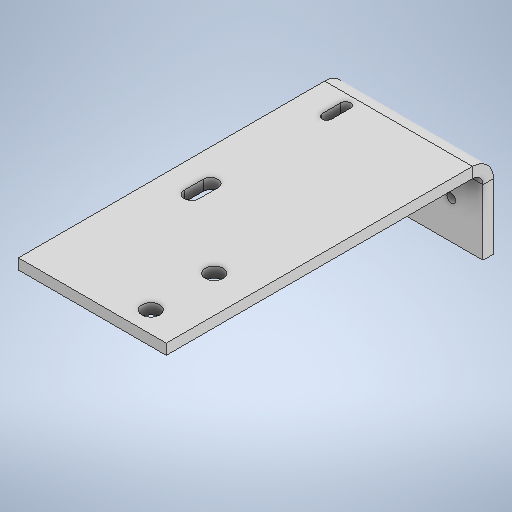
# Autodesk Inventor part: ER_Halterung_Kantensensor
Saved by Autodesk Inventor 2025.1 (Build 291241000, 241)
## iProperties
Created: 2025-06-20
Part Number: ER_Halterung_Kantensensor
Material: Generic
Document SubType Name: Sheet Metal
Designer: Erik
Density: 1 g/cm^3
Sheet Metal Rule: Default_mm
Appearance: Default
Author: Erik
Autodesk Inventor part; units mm, degrees
ref_plane "YZ Plane" through (0, 0, 0) normal (1, 0, 0) x (0, 1, 0)
ref_plane "XZ Plane" through (0, 0, 0) normal (0, 1, 0) x (-1, 0, 0)
ref_plane "XY Plane" through (0, 0, 0) normal (0, 0, 1) x (1, 0, 0)
sketch "Sketch1" plane through (0, 0, 0) normal (0, 1, 0) x (-1, 0, 0)
  line L0 (0, 0) -> (70, 0)
  line L1 (70, 0) -> (70, -150)
  line L2 (70, -150) -> (0, -150)
  line L3 (0, -150) -> (0, 0)
  dimension "d0" = 70
  dimension "d1" = 150
  measures "d0" distance of L1.end L2.end
  measures "d1" distance of L0.end L1.end
extrude "Plate1" add sketch "Sketch1" along normal blind 5
sketch "Sketch2" plane through (0, 0, -150) normal (0, 0, -1) x (-1, 0, 0)
  line L0 (70, 5) -> (0, 5)
  line L1 (0, 5) -> (70, 5)
  line L2 (70, 5) -> (70, -36)
  line L3 (70, -36) -> (0, -36)
  line L4 (0, -36) -> (0, 5)
  point P0 (0, 0)
  dimension "d3" = 70
  dimension "d4" = 41
  measures "d3" distance of L2.end L3.end
  measures "d4" distance of L1.end L2.end
sheet face with bend "Face2" sketch "Sketch2" thickness 5 toward (0, 0, -1) bend radius 5 relief straight relief width 5 relief depth 2.5
bend "Bend1"
sketch "Sketch3" plane through (0, 0, -155) normal (0, 0, -1) x (-1, 0, 0)
  line L0 (70, -36) -> (0, -36) projected
  line L1 (70, -5) -> (70, -36) projected
  point P0 (0, 0)
  point P1 (45, -18)
  point P2 (15, -18)
  dimension "d10" = 18
  dimension "d11" = 18
  dimension "d19" = 25
  dimension "d20" = 30
  measures "d10" distance from line of L0 point (45, -18)
  measures "d11" distance from line of L0 point (15, -18)
  measures "d19" distance from line of L1 point (45, -18)
  measures "d20" distance of point (45, -18) point (15, -18)
hole "Hole1" at (-45, -18, -155) at (-15, -18, -155) direction (0, 0, 1) diameter 4.134 depth 5 tip angle 118 thread size "M5x0.8" class "6H" standard "ISO Metric profile"
sketch "Sketch4" plane through (0, 5, 0) normal (0, 1, 0) x (1, 0, 0)
  line L0 (-70, 145) -> (0, 145) projected
  line L1 (-55, 145) -> (-55, 0) construction
  line L2 (-70, 0) -> (0, 0) projected
  line L3 (-70, 0) -> (-70, 145) projected
  line L4 (-57.25, 131) -> (-52.75, 131)
  line L5 (-52.75, 131) -> (-52.75, 140)
  line L6 (-52.75, 140) -> (-57.25, 140)
  line L7 (-57.25, 140) -> (-57.25, 131)
  line L8 (-57.25, 131) -> (-52.75, 140) construction
  line L9 (-52.75, 131) -> (-57.25, 140) construction
  arc A0 (-52.75, 140) -> (-57.25, 140) centre (-55, 140) ccw
  arc A1 (-57.25, 131) -> (-52.75, 131) centre (-55, 131) ccw
  line L10 (-55, 140) -> (-51.5, 76.0958) construction
  line L11 (-55, 140) -> (9, 140) construction
  line L12 (-55, 131) -> (-51.5, 67.0958) construction
  line L13 (-55, 131) -> (9, 131) construction
  line L14 (-58.5, 67) -> (-51.5, 67)
  line L15 (-51.5, 67) -> (-51.5, 76)
  line L16 (-51.5, 76) -> (-58.5, 76)
  line L17 (-58.5, 76) -> (-58.5, 67)
  line L18 (-58.5, 67) -> (-51.5, 76) construction
  line L19 (-51.5, 67) -> (-58.5, 76) construction
  arc A2 (-51.5, 76) -> (-58.5, 76) centre (-55, 76) ccw
  arc A3 (-58.5, 67) -> (-51.5, 67) centre (-55, 67) ccw
  point P0 (-70, 72.5)
  point P1 (-55, 135.5)
  point P2 (-55, 71.5)
  dimension "d21" = 15
  dimension "d22" = 4.5
  dimension "d23" = 9
  dimension "d25" = 5
  dimension "d32" = 64
  dimension "d34" = 64
  dimension "d36" = 7
  dimension "d37" = 9
  dimension "d40" = 64
  constraints: 34 end point, 8 midpoint, 8 point on circle, 8 tangent, 6 point on line, 4 centre point, 4 horizontal, 4 parallel, 2 equal length, 2 perpendicular, 1 vertical
  measures "d21" distance from line of point (-70, 72.5) L1
  measures "d22" distance between parallel lines of L5 L7
  measures "d23" distance of point (-55, 140) point (-55, 131)
  measures "d25" distance from line of L0 point (-55, 140)
  measures "d32" distance of L10.start L10.end
  measures "d34" distance of L12.start L12.end
  measures "d36" distance of L16.end L15.end
  measures "d37" distance between parallel lines of L16 L14
  measures "d40" distance of point (-55, 140) point (-55, 76)
extrude "Extrusion1" cut sketch "Sketch4" against normal up to surface (5 mm away)
sketch "Sketch5" plane through (0, 5, 0) normal (0, 1, 0) x (1, 0, 0)
  line L0 (-70, 0) -> (-70, 145) projected
  line L1 (0, 0) -> (-70, 0) projected
  point P0 (-17.3, 40)
  point P1 (-17.3, 10)
  dimension "d41" = 52.7
  dimension "d42" = 52.7
  dimension "d50" = 30
  dimension "d51" = 10
  measures "d41" distance from line of L0 point (-17.3, 40)
  measures "d42" distance from line of L0 point (-17.3, 10)
  measures "d50" distance of point (-17.3, 40) point (-17.3, 10)
  measures "d51" distance from line of L1 point (-17.3, 10)
hole "Hole2" at (-17.3, 5, -10) at (-17.3, 5, -40) direction (0, -1, 0) diameter 8.5 end through all
equation "\"d11\" = d10"
equation "\"d17\" = Thickness"
equation "\"d37\" = d23"
equation "\"d2\" = Thickness"
equation "\"d5\" = BendRadius"
equation "\"d6\" = BendReliefWidth"
equation "\"d8\" = MinimumRemnant"
equation "\"d7\" = BendReliefDepth"
equation "\"d9\" = TransitionRadius"
equation "\"d42\" = d41"
equation "\"BendRadius\" = Thickness"
equation "\"BendReliefWidth\" = Thickness"
equation "\"BendReliefDepth\" = 0.5 * Thickness"
equation "\"TransitionRadius\" = BendRadius"
equation "\"JacobiRadiusSize\" = BendRadius"
equation "\"GapSize\" = Thickness"
equation "\"Thickness\" = 5"
equation "\"MinimumRemnant\" = 10"
body "Solid1"
